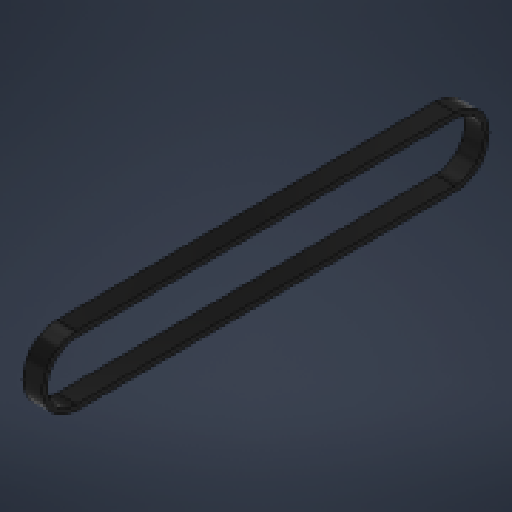
# Autodesk Inventor part: STANDIN,130T,HTD5mm,BELT
Saved by Autodesk Inventor 2026.1 (Build 301233020, 233B)
## iProperties
Created: 2026-01-29
Part Number: STANDIN,130T,HTD5mm,BELT
Material: Nylon 6/6
Document SubType Name: Modeling
Designer: Owen L
Density: 1.13 g/cm^3
Appearance: Smooth - Black
Author: Owen L
Autodesk Inventor part; units mm, degrees
ref_plane "YZ Plane" through (0, 0, 0) normal (1, 0, 0) x (0, 1, 0)
ref_plane "XZ Plane" through (0, 0, 0) normal (0, 1, 0) x (-1, 0, 0)
ref_plane "XY Plane" through (0, 0, 0) normal (0, 0, 1) x (1, 0, 0)
sketch "Sketch1" plane through (0, 0, 0) normal (1, 0, 0) x (0, 1, 0)
  arc A0 (-13.4131, 0) -> (13.4131, 0) centre (0, 0) ccw
  arc A1 (-15.9131, 0) -> (15.9131, 0) centre (0, 0) ccw
  arc A2 (13.4131, 175.006) -> (-13.4131, 175.006) centre (0, 175.006) ccw
  arc A3 (15.9131, 175.006) -> (-15.9131, 175.006) centre (0, 175.006) ccw
  line L0 (13.4131, 0) -> (13.4131, 175.006)
  line L1 (-13.4131, 0) -> (-13.4131, 175.006)
  line L2 (15.9131, 0) -> (15.9131, 175.006)
  line L3 (-15.9131, 0) -> (-15.9131, 175.006)
  dimension "d0" = 2.5
  dimension "d2" = 175.006
  dimension "d5" = 13.4131
  constraints: 9 end point, 9 horizontal alignment, 9 point on circle, 4 centre point, 4 vertical, 3 coincident, 1 vertical alignment
  measures "d0" radial gap between concentric circles of A1 A0
  measures "d2" distance of A2.centre point (0, 0)
  measures "d5" radius of A0
extrude "Extrusion1" add sketch "Sketch1" along normal blind 9
body "Solid1"
